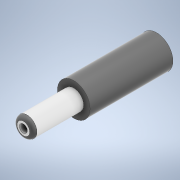
# Autodesk Inventor part: DC_PLUG
Saved by Autodesk Inventor 2020 (Build 240168000, 168)
## iProperties
Created: 2023-09-20
Part Number: DC_PLUG
Material: 일반
Document SubType Name: Modeling
Designer: ac837
Density: 1 g/cm^3
Appearance: 기본값
Author: ac837
Autodesk Inventor part; units mm, degrees
ref_plane "YZ Plane" through (0, 0, 0) normal (1, 0, 0) x (0, 1, 0)
ref_plane "XZ Plane" through (0, 0, 0) normal (0, 1, 0) x (-1, 0, 0)
ref_plane "XY Plane" through (0, 0, 0) normal (0, 0, 1) x (1, 0, 0)
sketch "스케치1" plane through (0, 0, 0) normal (0, 0, 1) x (1, 0, 0)
  circle A0 centre (0, 0) radius 2.725
  dimension "d0" = 5.45
  constraints: 1 centre point, 1 coincident
  measures "d0" diameter of A0
extrude "돌출1" add sketch "스케치1" along normal blind 13.8
sketch "스케치2" plane through (0, 0, 13.8) normal (0, 0, 1) x (1, 0, 0)
  circle A0 centre (0, 0) radius 1.075
  dimension "d3" = 2.15
  constraints: 1 centre point, 1 coincident
  measures "d3" diameter of A0
extrude "돌출2" cut sketch "스케치2" against normal blind 20.45
fillet "모깎기1" radius 1 1 edges at (-2.725, 0, 13.8)
sketch "스케치3" plane through (0, 0, 0) normal (0, 0, -1) x (-1, 0, 0)
  circle A0 centre (0, 0) radius 4.475
  dimension "d7" = 8.95
  constraints: 1 centre point, 1 coincident
  measures "d7" diameter of A0
extrude "돌출3" add sketch "스케치3" along normal blind 22.7
sketch "스케치4" plane through (0, 0, -22.7) normal (0, 0, -1) x (-1, 0, 0)
  circle A0 centre (0, 0) radius 1.075 projected
  circle A1 centre (0, 0) radius 3
  dimension "d10" = 6
  constraints: 1 centre point, 1 coincident
  measures "d10" diameter of A1
extrude "돌출4" cut sketch "스케치4" against normal blind 18.8 contours A0 | A1
